Autodesk Fusion 360 part; units mm, degrees
(part 7 of 25)
  arc A2762 (31.8052, 43.4657) -> (31.8052, 43.5293) centre (31.8052, 43.4975) ccw
  arc A2763 (9.9295, 17.8435) -> (9.866, 17.8435) centre (9.8978, 17.8435) ccw
  arc A2764 (11.39, 17.0815) -> (11.3265, 17.0815) centre (11.3582, 17.0815) ccw
  arc A2765 (9.866, 16.7005) -> (9.9295, 16.7005) centre (9.8978, 16.7005) ccw
  arc A2766 (30.353, 44.0055) -> (30.353, 44.6405) centre (30.353, 44.323) ccw
  arc A2767 (32.6942, 43.4657) -> (32.6942, 43.5293) centre (32.6942, 43.4975) ccw
  line L862 (9.5802, 16.7005) -> (10.2152, 16.7005)
  line L863 (10.7232, 17.018) -> (10.7232, 17.3355)
  line L864 (9.5802, 17.5895) -> (9.8977, 17.8435)
  arc A2768 (8.4773, 17.8435) -> (8.4138, 17.8435) centre (8.4456, 17.8435) ccw
  arc A2769 (9.5802, 16.7323) -> (9.5802, 16.6688) centre (9.5802, 16.7005) ccw
  line L865 (10.7232, 17.3355) -> (11.1042, 17.3355)
  line L866 (30.0355, 43.4975) -> (30.0355, 44.6405)
  line L867 (32.3132, 44.6405) -> (32.9482, 44.6405)
  arc A2770 (11.3265, 17.0815) -> (11.39, 17.0815) centre (11.3582, 17.0815) ccw
  arc A2771 (32.2815, 44.1325) -> (32.345, 44.1325) centre (32.3133, 44.1325) ccw
  arc A2772 (8.4138, 16.7005) -> (8.4773, 16.7005) centre (8.4456, 16.7005) ccw
  arc A2773 (30.353, 44.6088) -> (30.353, 44.6723) centre (30.353, 44.6406) ccw
  arc A2774 (32.3132, 44.6723) -> (32.3132, 44.6088) centre (32.3132, 44.6406) ccw
  arc A2775 (32.98, 43.8785) -> (32.9165, 43.8785) centre (32.9483, 43.8785) ccw
  arc A2776 (8.4455, 17.8753) -> (8.4455, 17.8118) centre (8.4455, 17.8436) ccw
  arc A2777 (32.9165, 43.8785) -> (32.98, 43.8785) centre (32.9483, 43.8785) ccw
  arc A2778 (32.6942, 44.1643) -> (32.6942, 44.1007) centre (32.6942, 44.1325) ccw
  arc A2779 (8.4455, 17.2402) -> (8.4455, 17.1768) centre (8.4455, 17.2085) ccw
  arc A2780 (9.9175, 17.8187) -> (9.8779, 17.8683) centre (9.8977, 17.8435) ccw
  arc A2781 (10.7232, 17.3672) -> (10.7232, 17.3038) centre (10.7232, 17.3355) ccw
  arc A2782 (32.3132, 43.5293) -> (32.3132, 43.4657) centre (32.3132, 43.4975) ccw
  arc A2783 (10.755, 17.018) -> (10.6915, 17.018) centre (10.7233, 17.018) ccw
  arc A2784 (10.755, 17.3355) -> (10.6915, 17.3355) centre (10.7233, 17.3355) ccw
  line L868 (8.4455, 16.7005) -> (8.4455, 17.8435)
  arc A2785 (32.9482, 43.8785) -> (32.6942, 44.1325) centre (32.6942, 43.8785) ccw
  line L869 (8.763, 17.2085) -> (8.4455, 17.2085)
  arc A2786 (32.9482, 44.6088) -> (32.9482, 44.6723) centre (32.9482, 44.6406) ccw
  line L870 (32.6942, 44.1325) -> (32.3132, 44.1325)
  line L871 (32.9482, 43.7515) -> (32.9482, 43.8785)
  line L872 (8.4455, 17.8435) -> (8.763, 17.8435)
  arc A2787 (8.763, 17.8753) -> (8.763, 17.8118) centre (8.763, 17.8436) ccw
  arc A2788 (10.2152, 16.6688) -> (10.2152, 16.7323) centre (10.2152, 16.7005) ccw
  arc A2789 (32.3132, 44.1643) -> (32.3132, 44.1007) centre (32.3132, 44.1325) ccw
  arc A2790 (11.3265, 17.018) -> (11.39, 17.018) centre (11.3582, 17.018) ccw
  arc A2791 (32.6942, 44.1007) -> (32.6942, 44.1643) centre (32.6942, 44.1325) ccw
  arc A2792 (10.7232, 17.018) -> (11.3582, 17.018) centre (11.0407, 17.018) ccw
  arc A2793 (8.763, 17.2402) -> (8.763, 17.1768) centre (8.763, 17.2085) ccw
  arc A2794 (8.763, 17.8118) -> (8.763, 17.8753) centre (8.763, 17.8436) ccw
  arc A2795 (11.2312, 17.8118) -> (11.2312, 17.8753) centre (11.2312, 17.8436) ccw
  line L873 (9.8977, 17.8435) -> (9.8977, 16.7005)
  arc A2796 (9.0521, 16.6863) -> (9.1089, 16.7147) centre (9.0805, 16.7005) ccw
  arc A2797 (82.4992, 5.1474) -> (82.5296, 5.2031) centre (82.5144, 5.1753) ccw
  arc A2798 (82.3595, 18.6055) -> (82.6135, 18.8595) centre (82.3595, 18.8595) ccw
  arc A2799 (82.4713, 19.0539) -> (82.5017, 19.1096) centre (82.4865, 19.0817) ccw
  arc A2800 (83.4326, 19.7168) -> (83.4327, 19.7802) centre (83.4326, 19.7485) ccw
  arc A2801 (83.0915, 5.6128) -> (83.1312, 5.5632) centre (83.1114, 5.588) ccw
  arc A2802 (82.5309, 19.6279) -> (82.5691, 19.6786) centre (82.55, 19.6532) ccw
  arc A2803 (82.1804, 5.3936) -> (82.15, 5.3379) centre (82.1652, 5.3657) ccw
  arc A2804 (82.5026, 19.1091) -> (82.4704, 19.0544) centre (82.4865, 19.0817) ccw
  line L874 (83.1113, 5.588) -> (83.4288, 5.842)
  arc A2805 (82.0699, 5.588) -> (82.0064, 5.588) centre (82.0382, 5.588) ccw
  line L875 (82.5144, 5.1753) -> (82.1652, 5.3658)
  arc A2806 (82.0064, 4.8578) -> (82.3874, 4.699) centre (82.3875, 5.2356) ccw
  arc A2807 (83.7463, 4.6673) -> (83.7463, 4.7307) centre (83.7463, 4.699) ccw
  arc A2808 (82.3595, 18.6372) -> (82.3595, 18.5738) centre (82.3595, 18.6055) ccw
  arc A2809 (83.4487, 5.8172) -> (83.409, 5.8668) centre (83.4289, 5.842) ccw
  arc A2810 (82.3874, 4.7307) -> (82.3874, 4.6673) centre (82.3874, 4.699) ccw
  arc A2811 (83.0592, 18.6261) -> (83.1076, 18.5849) centre (83.0834, 18.6055) ccw
  arc A2812 (82.6097, 4.953) -> (82.6732, 4.953) centre (82.6414, 4.953) ccw
  arc A2813 (82.2643, 19.7485) -> (82.0102, 19.4945) centre (82.2643, 19.4944) ccw
  arc A2814 (83.4327, 19.7802) -> (83.4327, 19.7168) centre (83.4327, 19.7485) ccw
  arc A2815 (83.7501, 19.4628) -> (83.6867, 19.4627) centre (83.7184, 19.4628) ccw
  arc A2816 (83.3971, 4.699) -> (83.4606, 4.699) centre (83.4288, 4.699) ccw
  arc A2817 (82.5779, 5.7468) -> (82.2922, 5.842) centre (82.2923, 5.3659) ccw
  arc A2818 (82.6453, 18.8595) -> (82.5817, 18.8595) centre (82.6135, 18.8595) ccw
  arc A2819 (82.55, 19.6532) -> (82.2643, 19.7485) centre (82.2642, 19.2724) ccw
  arc A2820 (82.2643, 19.7168) -> (82.2643, 19.7802) centre (82.2643, 19.7485) ccw
  line L876 (83.6232, 19.2405) -> (83.0834, 18.6055)
  arc A2821 (83.6473, 19.2199) -> (83.599, 19.2611) centre (83.6232, 19.2405) ccw
  arc A2822 (83.0834, 18.6372) -> (83.0834, 18.5738) centre (83.0834, 18.6055) ccw
  arc A2823 (82.1211, 19.2449) -> (82.1534, 19.2996) centre (82.1372, 19.2723) ccw
  arc A2824 (82.3595, 18.5738) -> (82.3595, 18.6372) centre (82.3595, 18.6055) ccw
  arc A2825 (83.0532, 19.5043) -> (83.1136, 19.4847) centre (83.0834, 19.4945) ccw
  arc A2826 (82.1491, 5.3384) -> (82.1813, 5.3931) centre (82.1652, 5.3658) ccw
  line L877 (83.0834, 18.6055) -> (83.7184, 18.6055)
  arc A2827 (82.029, 4.8801) -> (81.9839, 4.8354) centre (82.0065, 4.8577) ccw
  arc A2828 (82.2922, 5.8738) -> (82.2922, 5.8103) centre (82.2922, 5.842) ccw
  arc A2829 (83.4606, 5.842) -> (83.3971, 5.842) centre (83.4288, 5.842) ccw
  arc A2830 (10.6915, 17.018) -> (10.755, 17.018) centre (10.7233, 17.018) ccw
  arc A2831 (82.6732, 4.953) -> (82.6097, 4.953) centre (82.6414, 4.953) ccw
  arc A2832 (82.0064, 5.588) -> (82.0699, 5.588) centre (82.0382, 5.588) ccw
  arc A2833 (83.6013, 19.2635) -> (83.645, 19.2175) centre (83.6231, 19.2405) ccw
  arc A2834 (82.2642, 19.7802) -> (82.2643, 19.7168) centre (82.2643, 19.7485) ccw
  arc A2835 (83.7184, 18.5738) -> (83.7184, 18.6372) centre (83.7184, 18.6055) ccw
  line L878 (83.1113, 4.699) -> (83.7463, 4.699)
  arc A2836 (82.0382, 5.588) -> (82.1652, 5.3658) centre (82.2961, 5.588) ccw
  arc A2837 (82.001, 18.7866) -> (81.956, 18.7419) centre (81.9785, 18.7643) ccw
  arc A2838 (83.4327, 19.7485) -> (83.0834, 19.4945) centre (83.4327, 19.3814) ccw
  arc A2839 (81.9785, 19.4945) -> (82.042, 19.4945) centre (82.0103, 19.4945) ccw
  arc A2840 (82.5306, 5.2026) -> (82.4983, 5.1479) centre (82.5145, 5.1753) ccw
  arc A2841 (82.2922, 5.842) -> (82.0382, 5.588) centre (82.2922, 5.588) ccw
  line L879 (83.4288, 5.842) -> (83.4288, 4.699)
  arc A2842 (82.5589, 5.7214) -> (82.597, 5.7721) centre (82.5779, 5.7468) ccw
  arc A2843 (11.1042, 17.3672) -> (11.1042, 17.3038) centre (11.1042, 17.3355) ccw
  arc A2844 (82.3874, 4.6673) -> (82.3874, 4.7307) centre (82.3874, 4.699) ccw
  arc A2845 (81.9785, 18.7643) -> (82.3595, 18.6055) centre (82.3596, 19.1421) ccw
  arc A2846 (11.1042, 17.3038) -> (11.1042, 17.3672) centre (11.1042, 17.3355) ccw
  arc A2847 (83.6867, 19.4627) -> (83.7502, 19.4627) centre (83.7185, 19.4627) ccw
  arc A2848 (11.2312, 17.8435) -> (10.7232, 17.3355) centre (11.2312, 17.3355) ccw
  arc A2849 (11.3582, 17.0815) -> (11.1042, 17.3355) centre (11.1042, 17.0815) ccw
  arc A2850 (82.2922, 5.8103) -> (82.2922, 5.8738) centre (82.2922, 5.842) ccw
  arc A2851 (82.6414, 4.953) -> (82.5144, 5.1753) centre (82.3834, 4.953) ccw
  arc A2852 (83.1113, 4.7307) -> (83.1113, 4.6673) centre (83.1113, 4.699) ccw
  line L880 (82.4865, 19.0817) -> (82.1373, 19.2722)
  arc A2853 (15.326, 27.5496) -> (15.281, 27.5049) centre (15.3035, 27.5273) ccw
  arc A2854 (15.875, 28.4163) -> (15.5893, 28.5115) centre (15.5894, 28.0354) ccw
  line L881 (16.7005, 28.5115) -> (17.0815, 28.5115)
  arc A2855 (15.4461, 28.0079) -> (15.4784, 28.0626) centre (15.4623, 28.0352) ccw
  arc A2856 (16.4782, 27.6225) -> (16.4148, 27.6225) centre (16.4465, 27.6225) ccw
  arc A2857 (17.6078, 28.2823) -> (17.6474, 28.2327) centre (17.6276, 28.2575) ccw
  line L882 (20.3073, 36.1315) -> (20.6248, 36.3855)
  arc A2858 (16.891, 28.0353) -> (16.891, 27.9718) centre (16.891, 28.0036) ccw
  line L883 (17.6276, 27.3685) -> (18.2626, 27.3685)
  arc A2859 (17.0815, 27.3368) -> (17.0815, 27.4002) centre (17.0815, 27.3685) ccw
  arc A2860 (15.9068, 27.6225) -> (15.9703, 27.6225) centre (15.9386, 27.6225) ccw
  arc A2861 (16.7005, 28.5115) -> (16.4465, 28.2575) centre (16.7005, 28.2575) ccw
  arc A2862 (15.4775, 28.0631) -> (15.447, 28.0074) centre (15.4622, 28.0353) ccw
  arc A2863 (17.0815, 28.4798) -> (17.0815, 28.5433) centre (17.0815, 28.5115) ccw
  arc A2864 (82.042, 19.4945) -> (81.9785, 19.4945) centre (82.0103, 19.4945) ccw
  arc A2865 (82.6135, 18.8595) -> (82.4865, 19.0817) centre (82.3556, 18.8595) ccw
  arc A2866 (82.1525, 19.3001) -> (82.122, 19.2444) centre (82.1372, 19.2723) ccw
  arc A2867 (16.4782, 28.2575) -> (16.4148, 28.2575) centre (16.4465, 28.2575) ccw
  arc A2868 (15.5892, 28.5433) -> (15.5893, 28.4798) centre (15.5893, 28.5115) ccw
  arc A2869 (17.0815, 27.9718) -> (17.0815, 28.0353) centre (17.0815, 28.0036) ccw
  arc A2870 (18.2626, 27.3368) -> (18.2626, 27.4002) centre (18.2626, 27.3685) ccw
  line L884 (20.6248, 36.3855) -> (20.6248, 35.2425)
  arc A2871 (15.3035, 27.5273) -> (15.6845, 27.3685) centre (15.6846, 27.9051) ccw
  arc A2872 (16.7005, 27.4002) -> (16.7005, 27.3368) centre (16.7005, 27.3685) ccw
  arc A2873 (15.3035, 28.2575) -> (15.367, 28.2575) centre (15.3353, 28.2575) ccw
  arc A2874 (82.0102, 19.4945) -> (82.1373, 19.2722) centre (82.2682, 19.4945) ccw
  line L885 (16.891, 28.0035) -> (17.0815, 28.0035)
  arc A2875 (15.5893, 28.4798) -> (15.5893, 28.5433) centre (15.5893, 28.5115) ccw
  arc A2876 (82.5817, 18.8595) -> (82.6453, 18.8595) centre (82.6135, 18.8595) ccw
  arc A2877 (15.6845, 27.3368) -> (15.6845, 27.4002) centre (15.6845, 27.3685) ccw
  arc A2878 (83.6232, 19.2405) -> (83.7184, 19.4627) centre (83.4116, 19.4626) ccw
  line L886 (19.558, 35.2425) -> (19.558, 36.3855)
  line L887 (16.4465, 27.6225) -> (16.4465, 28.2575)
  line L888 (17.0815, 28.0035) -> (17.0815, 27.3685)
  arc A2879 (19.5263, 35.2425) -> (19.5897, 35.2425) centre (19.558, 35.2425) ccw
  arc A2880 (20.6446, 36.3607) -> (20.605, 36.4103) centre (20.6248, 36.3855) ccw
  arc A2881 (20.2875, 36.1563) -> (20.3271, 36.1067) centre (20.3073, 36.1315) ccw
  arc A2882 (16.4465, 27.6225) -> (16.7005, 27.3685) centre (16.7005, 27.6225) ccw
  arc A2883 (15.9703, 27.6225) -> (15.9068, 27.6225) centre (15.9386, 27.6225) ccw
  arc A2884 (15.8559, 28.3909) -> (15.8941, 28.4416) centre (15.875, 28.4163) ccw
  arc A2885 (83.7184, 19.4627) -> (83.4327, 19.7485) centre (83.4326, 19.4627) ccw
  arc A2886 (17.9134, 27.3685) -> (17.9768, 27.3685) centre (17.9451, 27.3685) ccw
  arc A2887 (16.7005, 27.3368) -> (16.7005, 27.4002) centre (16.7005, 27.3685) ccw
  arc A2888 (15.5893, 28.5115) -> (15.3353, 28.2575) centre (15.5893, 28.2575) ccw
  arc A2889 (17.9649, 28.4867) -> (17.9253, 28.5363) centre (17.9451, 28.5115) ccw
  arc A2890 (20.6565, 36.3855) -> (20.5931, 36.3855) centre (20.6248, 36.3855) ccw
  line L889 (17.9451, 28.5115) -> (17.9451, 27.3685)
  line L890 (19.2405, 36.3855) -> (19.8755, 36.3855)
  arc A2891 (16.7005, 28.4798) -> (16.7005, 28.5433) centre (16.7005, 28.5115) ccw
  arc A2892 (16.4148, 27.6225) -> (16.4782, 27.6225) centre (16.4465, 27.6225) ccw
  arc A2893 (17.0498, 27.3685) -> (17.1133, 27.3685) centre (17.0816, 27.3685) ccw
  arc A2894 (16.4148, 28.2575) -> (16.4782, 28.2575) centre (16.4465, 28.2575) ccw
  line L891 (17.0815, 27.3685) -> (16.7005, 27.3685)
  arc A2895 (15.6845, 27.4002) -> (15.6845, 27.3368) centre (15.6845, 27.3685) ccw
  arc A2896 (15.8276, 27.8721) -> (15.7954, 27.8174) centre (15.8115, 27.8448) ccw
  arc A2897 (15.3353, 28.2575) -> (15.4623, 28.0353) centre (15.5932, 28.2575) ccw
  arc A2898 (15.367, 28.2575) -> (15.3035, 28.2575) centre (15.3353, 28.2575) ccw
  line L892 (15.8115, 27.8448) -> (15.4623, 28.0353)
  arc A2899 (15.7963, 27.8169) -> (15.8267, 27.8726) centre (15.8115, 27.8448) ccw
  arc A2900 (17.1133, 28.0035) -> (17.0498, 28.0035) centre (17.0816, 28.0035) ccw
  arc A2901 (15.9385, 27.6225) -> (15.8115, 27.8448) centre (15.6805, 27.6225) ccw
  arc A2902 (16.7005, 28.5433) -> (16.7005, 28.4798) centre (16.7005, 28.5115) ccw
  line L893 (17.6276, 28.2575) -> (17.9451, 28.5115)
  arc A2903 (15.6845, 27.3685) -> (15.9385, 27.6225) centre (15.6845, 27.6225) ccw
  arc A2904 (17.6276, 27.4002) -> (17.6276, 27.3368) centre (17.6276, 27.3685) ccw
  arc A2905 (20.5931, 35.2425) -> (20.6565, 35.2425) centre (20.6248, 35.2425) ccw
  line L894 (20.3073, 35.2425) -> (20.9423, 35.2425)
  arc A2906 (17.9768, 28.5115) -> (17.9134, 28.5115) centre (17.9451, 28.5115) ccw
  arc A2907 (19.2405, 36.4173) -> (19.2405, 36.3537) centre (19.2405, 36.3855) ccw
  arc A2908 (19.5897, 36.3855) -> (19.5263, 36.3855) centre (19.558, 36.3855) ccw
  arc A2909 (20.3073, 35.2743) -> (20.3073, 35.2107) centre (20.3073, 35.2425) ccw
  arc A2910 (20.9423, 35.2107) -> (20.9423, 35.2743) centre (20.9423, 35.2425) ccw
  arc A2911 (19.8755, 36.3537) -> (19.8755, 36.4173) centre (19.8755, 36.3855) ccw
sketch "Botton Trace" plane through (0, 0, 0) normal (0, 0, 1) x (1, 0, 0)
  arc A0 (82.7578, 33.1788) -> (82.7578, 32.8613) centre (82.7578, 33.0201) ccw
  arc A1 (15.6337, 33.8137) -> (15.6337, 33.4963) centre (15.6337, 33.655) ccw
  arc A2 (82.4468, 33.8137) -> (82.4468, 33.4963) centre (82.4468, 33.655) ccw
  arc A3 (66.04, 33.1788) -> (66.04, 32.8613) centre (66.04, 33.0201) ccw
  arc A4 (81.28, 32.8613) -> (81.28, 33.1788) centre (81.28, 33.0201) ccw
  arc A5 (66.04, 33.4963) -> (66.04, 33.8137) centre (66.04, 33.655) ccw
  arc A6 (0.7747, 33.8137) -> (0.7747, 33.4963) centre (0.7747, 33.655) ccw
  arc A7 (52.818, 33.8137) -> (52.818, 33.4963) centre (52.818, 33.655) ccw
  arc A8 (15.7861, 33.4963) -> (15.7861, 33.8137) centre (15.7861, 33.655) ccw
  arc A9 (71.8947, 32.8613) -> (71.8947, 33.1788) centre (71.8947, 33.0201) ccw
  arc A10 (81.28, 33.8137) -> (81.28, 33.4963) centre (81.28, 33.655) ccw
  arc A11 (35.9156, 33.8137) -> (35.9156, 33.4963) centre (35.9156, 33.655) ccw
  arc A12 (39.1736, 33.4963) -> (39.1736, 33.8137) centre (39.1736, 33.655) ccw
  arc A13 (11.289, 33.8137) -> (11.289, 33.4963) centre (11.289, 33.655) ccw
  arc A14 (52.2859, 33.1788) -> (52.2859, 32.8613) centre (52.2859, 33.0201) ccw
  arc A15 (33.2611, 32.8613) -> (33.2611, 33.1788) centre (33.2611, 33.0201) ccw
  arc A16 (84.2253, 32.8613) -> (84.2253, 33.1788) centre (84.2253, 33.0201) ccw
  arc A17 (17.7419, 33.8137) -> (17.7419, 33.4963) centre (17.7419, 33.655) ccw
  arc A18 (35.3189, 33.1788) -> (35.3189, 32.8613) centre (35.3189, 33.0201) ccw
  arc A19 (31.002, 33.4963) -> (31.002, 33.8137) centre (31.002, 33.655) ccw
  arc A20 (48.6064, 33.1788) -> (48.6064, 32.8613) centre (48.6064, 33.0201) ccw
  arc A21 (17.7419, 33.1788) -> (17.7419, 32.8613) centre (17.7419, 33.0201) ccw
  arc A22 (49.3141, 32.8613) -> (49.3141, 33.1788) centre (49.3141, 33.0201) ccw
  arc A23 (54.9021, 32.8613) -> (54.9021, 33.1788) centre (54.9021, 33.0201) ccw
  arc A24 (84.2253, 33.4963) -> (84.2253, 33.8137) centre (84.2253, 33.655) ccw
  arc A25 (28.2956, 34.4487) -> (28.2956, 34.1313) centre (28.2956, 34.29) ccw
  arc A26 (0.7747, 35.0838) -> (0.7747, 34.7663) centre (0.7747, 34.925) ccw
  line L0 (61.7097, 34.29) -> (62.7503, 34.29)
  arc A27 (84.2253, 34.1313) -> (84.2253, 34.4487) centre (84.2253, 34.29) ccw
  arc A28 (72.517, 34.1313) -> (72.517, 34.4487) centre (72.517, 34.29) ccw
  arc A29 (61.7097, 34.4487) -> (61.7097, 34.1313) centre (61.7097, 34.29) ccw
  arc A30 (17.7419, 34.4487) -> (17.7419, 34.1313) centre (17.7419, 34.29) ccw
  arc A31 (79.7179, 34.4487) -> (79.7179, 34.1313) centre (79.7179, 34.29) ccw
  arc A32 (25.0444, 34.1313) -> (25.0444, 34.4487) centre (25.0444, 34.29) ccw
  arc A33 (56.974, 35.0838) -> (56.974, 34.7663) centre (56.974, 34.925) ccw
  arc A34 (57.1337, 34.4487) -> (57.1337, 34.1313) centre (57.1337, 34.29) ccw
  arc A35 (12.6332, 34.7663) -> (12.6332, 35.0838) centre (12.6332, 34.925) ccw
  arc A36 (60.2103, 34.1313) -> (60.2103, 34.4487) centre (60.2103, 34.29) ccw
  arc A37 (15.613, 34.4487) -> (15.613, 34.1313) centre (15.613, 34.29) ccw
  arc A38 (30.367, 34.1313) -> (30.367, 34.4487) centre (30.367, 34.29) ccw
  arc A39 (54.6263, 34.1313) -> (54.6263, 34.4487) centre (54.6263, 34.29) ccw
  arc A40 (39.8086, 34.1313) -> (39.8086, 34.4487) centre (39.8086, 34.29) ccw
  arc A41 (49.9686, 34.1313) -> (49.9686, 34.4487) centre (49.9686, 34.29) ccw
  arc A42 (35.9156, 34.4487) -> (35.9156, 34.1313) centre (35.9156, 34.29) ccw
  arc A43 (1.0423, 34.7663) -> (1.0423, 35.0838) centre (1.0423, 34.925) ccw
  arc A44 (53.453, 34.4487) -> (53.453, 34.1313) centre (53.453, 34.29) ccw
  arc A45 (62.7503, 34.1313) -> (62.7503, 34.4487) centre (62.7503, 34.29) ccw
  arc A46 (39.0236, 32.8613) -> (39.0236, 33.1788) centre (39.0236, 33.0201) ccw
  arc A47 (81.28, 33.1788) -> (81.28, 32.8613) centre (81.28, 33.0201) ccw
  arc A48 (79.7179, 35.0838) -> (79.7179, 34.7663) centre (79.7179, 34.925) ccw
  arc A49 (41.4714, 34.4487) -> (41.4714, 34.1313) centre (41.4714, 34.29) ccw
  arc A50 (72.517, 34.7663) -> (72.517, 35.0838) centre (72.517, 34.925) ccw
  arc A51 (54.088, 35.0838) -> (54.088, 34.7663) centre (54.088, 34.925) ccw
  arc A52 (10.654, 34.4487) -> (10.654, 34.1313) centre (10.654, 34.29) ccw
  arc A53 (84.2253, 34.7663) -> (84.2253, 35.0838) centre (84.2253, 34.925) ccw
  arc A54 (12.3063, 33.4963) -> (12.3063, 33.8137) centre (12.3063, 33.655) ccw
  arc A55 (15.7861, 34.7663) -> (15.7861, 35.0838) centre (15.7861, 34.925) ccw
  arc A56 (66.04, 32.8613) -> (66.04, 33.1788) centre (66.04, 33.0201) ccw
  arc A57 (25.0444, 33.4963) -> (25.0444, 33.8137) centre (25.0444, 33.655) ccw
  arc A58 (15.7861, 34.1313) -> (15.7861, 34.4487) centre (15.7861, 34.29) ccw
  arc A59 (25.6411, 32.8613) -> (25.6411, 33.1788) centre (25.6411, 33.0201) ccw
  arc A60 (56.8579, 33.1788) -> (56.8579, 32.8613) centre (56.8579, 33.0201) ccw
  arc A61 (0.9017, 34.1313) -> (0.9017, 34.4487) centre (0.9017, 34.29) ccw
  arc A62 (29.5021, 36.6713) -> (29.5021, 36.9887) centre (29.5021, 36.83) ccw
  arc A63 (72.214, 36.3537) -> (72.214, 36.0363) centre (72.214, 36.195) ccw
  arc A64 (4.5252, 35.7188) -> (4.5252, 35.4013) centre (4.5252, 35.5601) ccw
  arc A65 (15.7861, 35.4013) -> (15.7861, 35.7188) centre (15.7861, 35.5601) ccw
  arc A66 (6.6508, 35.4013) -> (6.6508, 35.7188) centre (6.6508, 35.5601) ccw
  arc A67 (72.517, 35.4013) -> (72.517, 35.7188) centre (72.517, 35.5601) ccw
  arc A68 (17.7419, 35.7188) -> (17.7419, 35.4013) centre (17.7419, 35.5601) ccw
  arc A69 (25.6411, 35.4013) -> (25.6411, 35.7188) centre (25.6411, 35.5601) ccw
  arc A70 (72.517, 36.0363) -> (72.517, 36.3537) centre (72.517, 36.195) ccw
  arc A71 (25.0444, 34.7663) -> (25.0444, 35.0838) centre (25.0444, 34.925) ccw
  arc A72 (51.322, 34.7663) -> (51.322, 35.0838) centre (51.322, 34.925) ccw
  arc A73 (27.6989, 36.9887) -> (27.6989, 36.6713) centre (27.6989, 36.83) ccw
  arc A74 (17.7419, 35.0838) -> (17.7419, 34.7663) centre (17.7419, 34.925) ccw
  arc A75 (29.732, 34.7663) -> (29.732, 35.0838) centre (29.732, 34.925) ccw
  arc A76 (64.2497, 34.4487) -> (64.2497, 34.1313) centre (64.2497, 34.29) ccw
  arc A77 (52.592, 36.0363) -> (52.592, 36.3537) centre (52.592, 36.195) ccw
  arc A78 (0.7747, 35.7188) -> (0.7747, 35.4013) centre (0.7747, 35.5601) ccw
  arc A79 (15.3068, 35.0838) -> (15.3068, 34.7663) centre (15.3068, 34.925) ccw
  arc A80 (35.9156, 35.0838) -> (35.9156, 34.7663) centre (35.9156, 34.925) ccw
  arc A81 (11.0836, 36.6713) -> (11.0836, 36.9887) centre (11.0836, 36.83) ccw
  arc A82 (84.2253, 35.4013) -> (84.2253, 35.7188) centre (84.2253, 35.5601) ccw
  arc A83 (14.3164, 36.9887) -> (14.3164, 36.6713) centre (14.3164, 36.83) ccw
  arc A84 (29.5021, 35.4013) -> (29.5021, 35.7188) centre (29.5021, 35.5601) ccw
  arc A85 (1.5708, 35.4013) -> (1.5708, 35.7188) centre (1.5708, 35.5601) ccw
  arc A86 (28.2956, 35.0838) -> (28.2956, 34.7663) centre (28.2956, 34.925) ccw
  arc A87 (29.5021, 36.0363) -> (29.5021, 36.3537) centre (29.5021, 36.195) ccw
  arc A88 (15.7861, 36.0363) -> (15.7861, 36.3537) centre (15.7861, 36.195) ccw
  arc A89 (10.1337, 35.0838) -> (10.1337, 34.7663) centre (10.1337, 34.925) ccw
  arc A90 (54.786, 34.7663) -> (54.786, 35.0838) centre (54.786, 34.925) ccw
  arc A91 (12.327, 34.1313) -> (12.327, 34.4487) centre (12.327, 34.29) ccw
  arc A92 (12.3536, 35.4013) -> (12.3536, 35.7188) centre (12.3536, 35.5601) ccw
  arc A93 (25.6921, 36.0363) -> (25.6921, 36.3537) centre (25.6921, 36.195) ccw
  arc A94 (17.7419, 36.3537) -> (17.7419, 36.0363) centre (17.7419, 36.195) ccw
  arc A95 (79.7179, 35.7188) -> (79.7179, 35.4013) centre (79.7179, 35.5601) ccw
  arc A96 (27.6989, 35.7188) -> (27.6989, 35.4013) centre (27.6989, 35.5601) ccw
  arc A97 (25.6411, 36.6713) -> (25.6411, 36.9887) centre (25.6411, 36.83) ccw
  arc A98 (15.113, 35.7188) -> (15.113, 35.4013) centre (15.113, 35.5601) ccw
  arc A99 (0.7747, 34.4487) -> (0.7747, 34.1313) centre (0.7747, 34.29) ccw
  arc A100 (27.6479, 36.3537) -> (27.6479, 36.0363) centre (27.6479, 36.195) ccw
  arc A101 (33.2611, 36.6713) -> (33.2611, 36.9887) centre (33.2611, 36.83) ccw
  arc A102 (0.7747, 36.3537) -> (0.7747, 36.0363) centre (0.7747, 36.195) ccw
  arc A103 (31.4579, 36.3537) -> (31.4579, 36.0363) centre (31.4579, 36.195) ccw
  arc A104 (84.2253, 36.0363) -> (84.2253, 36.3537) centre (84.2253, 36.195) ccw
  arc A105 (31.4579, 36.9887) -> (31.4579, 36.6713) centre (31.4579, 36.83) ccw
  arc A106 (35.3189, 36.9887) -> (35.3189, 36.6713) centre (35.3189, 36.83) ccw
  arc A107 (17.7419, 36.9887) -> (17.7419, 36.6713) centre (17.7419, 36.83) ccw
  arc A108 (51.6314, 36.9887) -> (51.6314, 36.6713) centre (51.6314, 36.83) ccw
  arc A109 (51.957, 35.4013) -> (51.957, 35.7188) centre (51.957, 35.5601) ccw
  arc A110 (79.7179, 36.3537) -> (79.7179, 36.0363) centre (79.7179, 36.195) ccw
  arc A111 (31.863, 35.7188) -> (31.863, 35.4013) centre (31.863, 35.5601) ccw
  arc A112 (9.6052, 35.7188) -> (9.6052, 35.4013) centre (9.6052, 35.5601) ccw
  arc A113 (72.214, 37.6238) -> (72.214, 37.3063) centre (72.214, 37.4651) ccw
  arc A114 (20.32, 37.9413) -> (20.32, 38.2587) centre (20.32, 38.1) ccw
  arc A115 (39.8086, 36.6713) -> (39.8086, 36.9887) centre (39.8086, 36.83) ccw
  arc A116 (33.2611, 35.4013) -> (33.2611, 35.7188) centre (33.2611, 35.5601) ccw
  arc A117 (0.7747, 36.9887) -> (0.7747, 36.6713) centre (0.7747, 36.83) ccw
  arc A118 (31.4579, 37.6238) -> (31.4579, 37.3063) centre (31.4579, 37.4651) ccw
  arc A119 (84.2253, 36.6713) -> (84.2253, 36.9887) centre (84.2253, 36.83) ccw
  arc A120 (18.6006, 37.3063) -> (18.6006, 37.6238) centre (18.6006, 37.4651) ccw
  arc A121 (79.7179, 36.9887) -> (79.7179, 36.6713) centre (79.7179, 36.83) ccw
  arc A122 (17.7419, 37.6238) -> (17.7419, 37.3063) centre (17.7419, 37.4651) ccw
  arc A123 (25.0444, 37.3063) -> (25.0444, 37.6238) centre (25.0444, 37.4651) ccw
  arc A124 (0.7747, 38.2587) -> (0.7747, 37.9413) centre (0.7747, 38.1) ccw
  arc A125 (3.4636, 37.9413) -> (3.4636, 38.2587) centre (3.4636, 38.1) ccw
  arc A126 (28.2956, 37.6238) -> (28.2956, 37.3063) centre (28.2956, 37.4651) ccw
  arc A127 (13.6814, 37.6238) -> (13.6814, 37.3063) centre (13.6814, 37.4651) ccw
  arc A128 (39.1736, 37.3063) -> (39.1736, 37.6238) centre (39.1736, 37.4651) ccw
  arc A129 (15.7861, 36.6713) -> (15.7861, 36.9887) centre (15.7861, 36.83) ccw
  arc A130 (17.7419, 38.2587) -> (17.7419, 37.9413) centre (17.7419, 38.1) ccw
  arc A131 (72.517, 36.6713) -> (72.517, 36.9887) centre (72.517, 36.83) ccw
  arc A132 (20.32, 37.6238) -> (20.32, 37.3063) centre (20.32, 37.4651) ccw
  arc A133 (35.3189, 35.7188) -> (35.3189, 35.4013) centre (35.3189, 35.5601) ccw
  arc A134 (49.9686, 36.6713) -> (49.9686, 36.9887) centre (49.9686, 36.83) ccw
  arc A135 (4.0986, 37.3063) -> (4.0986, 37.6238) centre (4.0986, 37.4651) ccw
  arc A136 (22.0394, 37.6238) -> (22.0394, 37.3063) centre (22.0394, 37.4651) ccw
  arc A137 (11.7186, 36.0363) -> (11.7186, 36.3537) centre (11.7186, 36.195) ccw
  arc A138 (20.32, 37.3063) -> (20.32, 37.6238) centre (20.32, 37.4651) ccw
  arc A139 (20.32, 38.2587) -> (20.32, 37.9413) centre (20.32, 38.1) ccw
  arc A140 (15.7861, 37.9413) -> (15.7861, 38.2587) centre (15.7861, 38.1) ccw
  arc A141 (72.3737, 36.9887) -> (72.3737, 36.6713) centre (72.3737, 36.83) ccw
  arc A142 (41.4714, 36.9887) -> (41.4714, 36.6713) centre (41.4714, 36.83) ccw
  arc A143 (15.7861, 37.3063) -> (15.7861, 37.6238) centre (15.7861, 37.4651) ccw
  arc A144 (53.227, 36.6713) -> (53.227, 36.9887) centre (53.227, 36.83) ccw
  arc A145 (54.723, 35.7188) -> (54.723, 35.4013) centre (54.723, 35.5601) ccw
  arc A146 (14.9442, 36.3537) -> (14.9442, 36.0363) centre (14.9442, 36.195) ccw
  arc A147 (13.0464, 38.2587) -> (13.0464, 37.9413) centre (13.0464, 38.1) ccw
  arc A148 (25.0444, 37.9413) -> (25.0444, 38.2587) centre (25.0444, 38.1) ccw
  arc A149 (29.5021, 37.9413) -> (29.5021, 38.2587) centre (29.5021, 38.1) ccw
  arc A150 (0.7747, 37.6238) -> (0.7747, 37.3063) centre (0.7747, 37.4651) ccw
  arc A151 (49.3336, 38.5763) -> (49.3336, 38.8937) centre (49.3336, 38.735) ccw
  arc A152 (84.2253, 38.5763) -> (84.2253, 38.8937) centre (84.2253, 38.735) ccw
  arc A153 (0.7747, 39.5288) -> (0.7747, 39.2113) centre (0.7747, 39.37) ccw
  arc A154 (72.517, 38.5763) -> (72.517, 38.8937) centre (72.517, 38.735) ccw
  arc A155 (2.8286, 38.5763) -> (2.8286, 38.8937) centre (2.8286, 38.735) ccw
  arc A156 (18.6006, 38.5763) -> (18.6006, 38.8937) centre (18.6006, 38.735) ccw
  arc A157 (79.7179, 38.2587) -> (79.7179, 37.9413) centre (79.7179, 38.1) ccw
  arc A158 (15.7861, 38.5763) -> (15.7861, 38.8937) centre (15.7861, 38.735) ccw
  arc A159 (12.4114, 38.8937) -> (12.4114, 38.5763) centre (12.4114, 38.735) ccw
  arc A160 (2.1936, 39.2113) -> (2.1936, 39.5288) centre (2.1936, 39.37) ccw
  arc A161 (37.578, 37.6238) -> (37.578, 37.3063) centre (37.578, 37.4651) ccw
  arc A162 (49.3336, 37.3063) -> (49.3336, 37.6238) centre (49.3336, 37.4651) ccw
  arc A163 (17.7419, 38.8937) -> (17.7419, 38.5763) centre (17.7419, 38.735) ccw
  arc A164 (21.7972, 39.5288) -> (21.7972, 39.2113) centre (21.7972, 39.37) ccw
  arc A165 (28.2956, 38.8937) -> (28.2956, 38.5763) centre (28.2956, 38.735) ccw
  arc A166 (42.2564, 38.2587) -> (42.2564, 37.9413) centre (42.2564, 38.1) ccw
  arc A167 (38.213, 38.2587) -> (38.213, 37.9413) centre (38.213, 38.1) ccw
  arc A168 (39.1541, 37.9413) -> (39.1541, 38.2587) centre (39.1541, 38.1) ccw
  arc A169 (28.2956, 38.2587) -> (28.2956, 37.9413) centre (28.2956, 38.1) ccw
  arc A170 (27.6989, 39.5288) -> (27.6989, 39.2113) centre (27.6989, 39.37) ccw
  arc A171 (18.8428, 39.2113) -> (18.8428, 39.5288) centre (18.8428, 39.37) ccw
  arc A172 (84.2253, 37.3063) -> (84.2253, 37.6238) centre (84.2253, 37.4651) ccw
  arc A173 (53.862, 37.3063) -> (53.862, 37.6238) centre (53.862, 37.4651) ccw
  arc A174 (32.6644, 37.3063) -> (32.6644, 37.6238) centre (32.6644, 37.4651) ccw
  arc A175 (33.2611, 39.2113) -> (33.2611, 39.5288) centre (33.2611, 39.37) ccw
  arc A176 (22.0394, 38.8937) -> (22.0394, 38.5763) centre (22.0394, 38.735) ccw
  arc A177 (38.848, 38.8937) -> (38.848, 38.5763) centre (38.848, 38.735) ccw
  arc A178 (29.5021, 37.3063) -> (29.5021, 37.6238) centre (29.5021, 37.4651) ccw
  arc A179 (32.6644, 37.9413) -> (32.6644, 38.2587) centre (32.6644, 38.1) ccw
  arc A180 (84.2253, 37.9413) -> (84.2253, 38.2587) centre (84.2253, 38.1) ccw
  arc A181 (42.8914, 38.8937) -> (42.8914, 38.5763) centre (42.8914, 38.735) ccw
  arc A182 (25.0444, 38.5763) -> (25.0444, 38.8937) centre (25.0444, 38.735) ccw
  arc A183 (79.7179, 38.8937) -> (79.7179, 38.5763) centre (79.7179, 38.735) ccw
  arc A184 (25.6411, 39.2113) -> (25.6411, 39.5288) centre (25.6411, 39.37) ccw
  arc A185 (42.1064, 37.6238) -> (42.1064, 37.3063) centre (42.1064, 37.4651) ccw
  arc A186 (79.7179, 37.6238) -> (79.7179, 37.3063) centre (79.7179, 37.4651) ccw
  arc A187 (72.214, 38.8937) -> (72.214, 38.5763) centre (72.214, 38.735) ccw
  arc A188 (52.2664, 37.6238) -> (52.2664, 37.3063) centre (52.2664, 37.4651) ccw
  arc A189 (29.5021, 38.5763) -> (29.5021, 38.8937) centre (29.5021, 38.735) ccw
  arc A190 (72.517, 37.3063) -> (72.517, 37.6238) centre (72.517, 37.4651) ccw
  arc A191 (31.4579, 38.8937) -> (31.4579, 38.5763) centre (31.4579, 38.735) ccw
  arc A192 (39.1736, 38.5763) -> (39.1736, 38.8937) centre (39.1736, 38.735) ccw
  arc A193 (18.3143, 39.8463) -> (18.3143, 40.1638) centre (18.3143, 40.0051) ccw
  arc A194 (32.6644, 38.5763) -> (32.6644, 38.8937) centre (32.6644, 38.735) ccw
  arc A195 (40.9286, 39.8463) -> (40.9286, 40.1638) centre (40.9286, 40.0051) ccw
  arc A196 (5.4264, 39.5288) -> (5.4264, 39.2113) centre (5.4264, 39.37) ccw
  arc A197 (49.3141, 37.9413) -> (49.3141, 38.2587) centre (49.3141, 38.1) ccw
  arc A198 (27.5014, 40.7987) -> (27.5014, 40.4813) centre (27.5014, 40.64) ccw
  arc A199 (72.517, 39.2113) -> (72.517, 39.5288) centre (72.517, 39.37) ccw
  arc A200 (17.7419, 39.5288) -> (17.7419, 39.2113) centre (17.7419, 39.37) ccw
  arc A201 (31.4579, 40.1638) -> (31.4579, 39.8463) centre (31.4579, 40.0051) ccw
  arc A202 (4.5252, 40.7987) -> (4.5252, 40.4813) centre (4.5252, 40.64) ccw
  arc A203 (29.5021, 40.4813) -> (29.5021, 40.7987) centre (29.5021, 40.64) ccw
  arc A204 (35.3189, 39.5288) -> (35.3189, 39.2113) centre (35.3189, 39.37) ccw
  arc A205 (84.2253, 39.2113) -> (84.2253, 39.5288) centre (84.2253, 39.37) ccw
  arc A206 (39.8086, 39.2113) -> (39.8086, 39.5288) centre (39.8086, 39.37) ccw
  arc A207 (9.6052, 40.7987) -> (9.6052, 40.4813) centre (9.6052, 40.64) ccw
  arc A208 (31.4579, 40.7987) -> (31.4579, 40.4813) centre (31.4579, 40.64) ccw
  arc A209 (52.2859, 38.2587) -> (52.2859, 37.9413) centre (52.2859, 38.1) ccw
  arc A210 (72.517, 37.9413) -> (72.517, 38.2587) centre (72.517, 38.1) ccw
  arc A211 (17.7419, 40.1638) -> (17.7419, 39.8463) centre (17.7419, 40.0051) ccw
  arc A212 (26.148, 40.1638) -> (26.148, 39.8463) centre (26.148, 40.0051) ccw
  arc A213 (37.987, 40.4813) -> (37.987, 40.7987) centre (37.987, 40.64) ccw
  arc A214 (49.9686, 39.2113) -> (49.9686, 39.5288) centre (49.9686, 39.37) ccw
  arc A215 (4.7914, 40.1638) -> (4.7914, 39.8463) centre (4.7914, 40.0051) ccw
  arc A216 (37.352, 39.8463) -> (37.352, 40.1638) centre (37.352, 40.0051) ccw
  arc A217 (31.4579, 38.2587) -> (31.4579, 37.9413) centre (31.4579, 38.1) ccw
  arc A218 (79.7179, 39.5288) -> (79.7179, 39.2113) centre (79.7179, 39.37) ccw
  arc A219 (1.905, 39.8463) -> (1.905, 40.1638) centre (1.905, 40.0051) ccw
  arc A220 (0.7747, 40.1638) -> (0.7747, 39.8463) centre (0.7747, 40.0051) ccw
  arc A221 (72.214, 40.1638) -> (72.214, 39.8463) centre (72.214, 40.0051) ccw
  arc A222 (15.7861, 39.2113) -> (15.7861, 39.5288) centre (15.7861, 39.37) ccw
  arc A223 (18.1737, 40.4813) -> (18.1737, 40.7987) centre (18.1737, 40.64) ccw
  arc A224 (35.9986, 40.4813) -> (35.9986, 40.7987) centre (35.9986, 40.64) ccw
  arc A225 (39.483, 39.5288) -> (39.483, 39.2113) centre (39.483, 39.37) ccw
  arc A226 (0.7747, 38.8937) -> (0.7747, 38.5763) centre (0.7747, 38.735) ccw
  arc A227 (17.7419, 40.7987) -> (17.7419, 40.4813) centre (17.7419, 40.64) ccw
  arc A228 (29.5021, 39.2113) -> (29.5021, 39.5288) centre (29.5021, 39.37) ccw
  arc A229 (72.3737, 39.5288) -> (72.3737, 39.2113) centre (72.3737, 39.37) ccw
  arc A230 (50.5114, 40.1638) -> (50.5114, 39.8463) centre (50.5114, 40.0051) ccw
  arc A231 (37.6614, 40.7987) -> (37.6614, 40.4813) centre (37.6614, 40.64) ccw
  arc A232 (36.717, 39.2113) -> (36.717, 39.5288) centre (36.717, 39.37) ccw
  arc A233 (43.5264, 39.5288) -> (43.5264, 39.2113) centre (43.5264, 39.37) ccw
  arc A234 (42.1986, 41.1163) -> (42.1986, 41.4337) centre (42.1986, 41.275) ccw
  arc A235 (66.04, 41.4337) -> (66.04, 41.1163) centre (66.04, 41.275) ccw
  arc A236 (29.5021, 39.8463) -> (29.5021, 40.1638) centre (29.5021, 40.0051) ccw
  arc A237 (18.8428, 41.7513) -> (18.8428, 42.0688) centre (18.8428, 41.9101) ccw
  arc A238 (79.7179, 40.1638) -> (79.7179, 39.8463) centre (79.7179, 40.0051) ccw
  arc A239 (0.7747, 41.4337) -> (0.7747, 41.1163) centre (0.7747, 41.275) ccw
  arc A240 (38.2964, 41.4337) -> (38.2964, 41.1163) centre (38.2964, 41.275) ccw
  arc A241 (72.517, 39.8463) -> (72.517, 40.1638) centre (72.517, 40.0051) ccw
  arc A242 (60.2103, 40.4813) -> (60.2103, 40.7987) centre (60.2103, 40.64) ccw
  arc A243 (62.7503, 40.4813) -> (62.7503, 40.7987) centre (62.7503, 40.64) ccw
  arc A244 (51.6314, 40.7987) -> (51.6314, 40.4813) centre (51.6314, 40.64) ccw
  arc A245 (51.322, 39.8463) -> (51.322, 40.1638) centre (51.322, 40.0051) ccw
  arc A246 (31.4579, 39.5288) -> (31.4579, 39.2113) centre (31.4579, 39.37) ccw
  arc A247 (64.2497, 40.7987) -> (64.2497, 40.4813) centre (64.2497, 40.64) ccw
  arc A248 (72.517, 41.1163) -> (72.517, 41.4337) centre (72.517, 41.275) ccw
  arc A249 (5.0537, 41.4337) -> (5.0537, 41.1163) centre (5.0537, 41.275) ccw
  arc A250 (79.7179, 40.7987) -> (79.7179, 40.4813) centre (79.7179, 40.64) ccw
  arc A251 (42.1064, 41.4337) -> (42.1064, 41.1163) centre (42.1064, 41.275) ccw
  arc A252 (28.1364, 41.4337) -> (28.1364, 41.1163) centre (28.1364, 41.275) ccw
  arc A253 (59.1697, 40.7987) -> (59.1697, 40.4813) centre (59.1697, 40.64) ccw
  arc A254 (6.6508, 40.4813) -> (6.6508, 40.7987) centre (6.6508, 40.64) ccw
  arc A255 (72.517, 40.4813) -> (72.517, 40.7987) centre (72.517, 40.64) ccw
  arc A256 (56.9091, 41.1163) -> (56.9091, 41.4337) centre (56.9091, 41.275) ccw
  arc A257 (6.1223, 41.1163) -> (6.1223, 41.4337) centre (6.1223, 41.275) ccw
  arc A258 (15.7861, 40.4813) -> (15.7861, 40.7987) centre (15.7861, 40.64) ccw
  arc A259 (66.04, 41.1163) -> (66.04, 41.4337) centre (66.04, 41.275) ccw
  arc A260 (15.7861, 41.7513) -> (15.7861, 42.0688) centre (15.7861, 41.9101) ccw
  arc A261 (10.908, 41.4337) -> (10.908, 41.1163) centre (10.908, 41.275) ccw
  arc A262 (61.7097, 40.7987) -> (61.7097, 40.4813) centre (61.7097, 40.64) ccw
  arc A263 (15.7861, 41.1163) -> (15.7861, 41.4337) centre (15.7861, 41.275) ccw
  arc A264 (1.5708, 40.4813) -> (1.5708, 40.7987) centre (1.5708, 40.64) ccw
  arc A265 (1.0423, 41.1163) -> (1.0423, 41.4337) centre (1.0423, 41.275) ccw
  arc A266 (84.2253, 39.8463) -> (84.2253, 40.1638) centre (84.2253, 40.0051) ccw
  arc A267 (41.5636, 40.4813) -> (41.5636, 40.7987) centre (41.5636, 40.64) ccw
  arc A268 (5.1943, 42.0688) -> (5.1943, 41.7513) centre (5.1943, 41.9101) ccw
  arc A269 (0.7747, 40.7987) -> (0.7747, 40.4813) centre (0.7747, 40.64) ccw
  arc A270 (15.7861, 39.8463) -> (15.7861, 40.1638) centre (15.7861, 40.0051) ccw
  arc A271 (11.543, 42.0688) -> (11.543, 41.7513) centre (11.543, 41.9101) ccw
  arc A272 (84.2253, 40.4813) -> (84.2253, 40.7987) centre (84.2253, 40.64) ccw
  arc A273 (17.7419, 41.4337) -> (17.7419, 41.1163) centre (17.7419, 41.275) ccw
  arc A274 (35.3636, 41.1163) -> (35.3636, 41.4337) centre (35.3636, 41.275) ccw
  arc A275 (40.118, 40.1638) -> (40.118, 39.8463) centre (40.118, 40.0051) ccw
  arc A276 (41.4714, 40.7987) -> (41.4714, 40.4813) centre (41.4714, 40.64) ccw
  arc A277 (18.3143, 41.1163) -> (18.3143, 41.4337) centre (18.3143, 41.275) ccw
  arc A278 (66.04, 42.7037) -> (66.04, 42.3863) centre (66.04, 42.545) ccw
  arc A279 (81.28, 42.3863) -> (81.28, 42.7037) centre (81.28, 42.545) ccw
  arc A280 (39.1736, 42.3863) -> (39.1736, 42.7037) centre (39.1736, 42.545) ccw
  arc A281 (38.2964, 42.7037) -> (38.2964, 42.3863) centre (38.2964, 42.545) ccw
  arc A282 (28.1559, 42.0688) -> (28.1559, 41.7513) centre (28.1559, 41.9101) ccw
  arc A283 (31.4579, 41.4337) -> (31.4579, 41.1163) centre (31.4579, 41.275) ccw
  arc A284 (32.498, 42.7037) -> (32.498, 42.3863) centre (32.498, 42.545) ccw
  arc A285 (42.658, 42.7037) -> (42.658, 42.3863) centre (42.658, 42.545) ccw
  arc A286 (25.1841, 41.7513) -> (25.1841, 42.0688) centre (25.1841, 41.9101) ccw
  arc A287 (72.517, 41.7513) -> (72.517, 42.0688) centre (72.517, 41.9101) ccw
  arc A288 (57.6703, 40.4813) -> (57.6703, 40.7987) centre (57.6703, 40.64) ccw
  arc A289 (29.732, 42.3863) -> (29.732, 42.7037) centre (29.732, 42.545) ccw
  arc A290 (67.2068, 41.4337) -> (67.2068, 41.1163) centre (67.2068, 41.275) ccw
  arc A291 (0.9017, 41.7513) -> (0.9017, 42.0688) centre (0.9017, 41.9101) ccw
  arc A292 (29.5021, 41.7513) -> (29.5021, 42.0688) centre (29.5021, 41.9101) ccw
  arc A293 (79.7179, 42.0688) -> (79.7179, 41.7513) centre (79.7179, 41.9101) ccw
  arc A294 (31.863, 42.0688) -> (31.863, 41.7513) centre (31.863, 41.9101) ccw
  arc A295 (84.2253, 41.7513) -> (84.2253, 42.0688) centre (84.2253, 41.9101) ccw
  arc A296 (5.0537, 42.7037) -> (5.0537, 42.3863) centre (5.0537, 42.545) ccw
  arc A297 (13.3018, 42.3863) -> (13.3018, 42.7037) centre (13.3018, 42.545) ccw
  arc A298 (66.04, 42.3863) -> (66.04, 42.7037) centre (66.04, 42.545) ccw
  arc A299 (42.1259, 42.0688) -> (42.1259, 41.7513) centre (42.1259, 41.9101) ccw
  arc A300 (17.7419, 42.7037) -> (17.7419, 42.3863) centre (17.7419, 42.545) ccw
  arc A301 (0.7747, 42.7037) -> (0.7747, 42.3863) centre (0.7747, 42.545) ccw
  arc A302 (79.7179, 41.4337) -> (79.7179, 41.1163) centre (79.7179, 41.275) ccw
  arc A303 (52.2664, 41.4337) -> (52.2664, 41.1163) centre (52.2664, 41.275) ccw
  arc A304 (0.7747, 42.0688) -> (0.7747, 41.7513) centre (0.7747, 41.9101) ccw
  arc A305 (35.3441, 41.7513) -> (35.3441, 42.0688) centre (35.3441, 41.9101) ccw
  arc A306 (81.28, 42.7037) -> (81.28, 42.3863) centre (81.28, 42.545) ccw
  arc A307 (21.7972, 42.0688) -> (21.7972, 41.7513) centre (21.7972, 41.9101) ccw
  arc A308 (15.7861, 42.3863) -> (15.7861, 42.7037) centre (15.7861, 42.545) ccw
  arc A309 (1.0423, 42.3863) -> (1.0423, 42.7037) centre (1.0423, 42.545) ccw
  arc A310 (67.5513, 42.7037) -> (67.5513, 42.3863) centre (67.5513, 42.545) ccw
  arc A311 (5.9817, 41.7513) -> (5.9817, 42.0688) centre (5.9817, 41.9101) ccw
  arc A312 (66.04, 41.7513) -> (66.04, 42.0688) centre (66.04, 41.9101) ccw
  arc A313 (49.3336, 42.3863) -> (49.3336, 42.7037) centre (49.3336, 42.545) ccw
  arc A314 (38.3159, 42.0688) -> (38.3159, 41.7513) centre (38.3159, 41.9101) ccw
  arc A315 (84.2253, 41.1163) -> (84.2253, 41.4337) centre (84.2253, 41.275) ccw
  arc A316 (28.1364, 42.7037) -> (28.1364, 42.3863) centre (28.1364, 42.545) ccw
  arc A317 (52.4164, 42.0688) -> (52.4164, 41.7513) centre (52.4164, 41.9101) ccw
  arc A318 (56.6547, 41.7513) -> (56.6547, 42.0688) centre (56.6547, 41.9101) ccw
  arc A319 (29.5021, 41.1163) -> (29.5021, 41.4337) centre (29.5021, 41.275) ccw
  arc A320 (38.622, 41.1163) -> (38.622, 41.4337) centre (38.622, 41.275) ccw
  arc A321 (72.1491, 42.3863) -> (72.1491, 42.7037) centre (72.1491, 42.545) ccw
  arc A322 (39.1541, 41.7513) -> (39.1541, 42.0688) centre (39.1541, 41.9101) ccw
  arc A323 (12.178, 42.7037) -> (12.178, 42.3863) centre (12.178, 42.545) ccw
  arc A324 (66.04, 43.6563) -> (66.04, 43.9738) centre (66.04, 43.815) ccw
  arc A325 (43.293, 43.3387) -> (43.293, 43.0213) centre (43.293, 43.18) ccw
  arc A326 (17.7419, 43.3387) -> (17.7419, 43.0213) centre (17.7419, 43.18) ccw
  arc A327 (15.4025, 43.3387) -> (15.4025, 43.0213) centre (15.4025, 43.18) ccw
  arc A328 (14.6382, 42.7037) -> (14.6382, 42.3863) centre (14.6382, 42.545) ccw
  arc A329 (15.7861, 43.0213) -> (15.7861, 43.3387) centre (15.7861, 43.18) ccw
  arc A330 (25.2036, 42.3863) -> (25.2036, 42.7037) centre (25.2036, 42.545) ccw
  arc A331 (41.162, 43.6563) -> (41.162, 43.9738) centre (41.162, 43.815) ccw
  arc A332 (81.28, 43.6563) -> (81.28, 43.9738) centre (81.28, 43.815) ccw
  arc A333 (84.2253, 43.0213) -> (84.2253, 43.3387) centre (84.2253, 43.18) ccw
  arc A334 (66.04, 43.9738) -> (66.04, 43.6563) centre (66.04, 43.815) ccw
  arc A335 (27.5014, 43.3387) -> (27.5014, 43.0213) centre (27.5014, 43.18) ccw
  arc A336 (18.1737, 43.0213) -> (18.1737, 43.3387) centre (18.1737, 43.18) ccw
  arc A337 (35.9986, 43.0213) -> (35.9986, 43.3387) centre (35.9986, 43.18) ccw
  arc A338 (31.002, 43.6563) -> (31.002, 43.9738) centre (31.002, 43.815) ccw
  arc A339 (0.7747, 43.3387) -> (0.7747, 43.0213) centre (0.7747, 43.18) ccw
  arc A340 (35.3636, 42.3863) -> (35.3636, 42.7037) centre (35.3636, 42.545) ccw
  arc A341 (81.28, 43.0213) -> (81.28, 43.3387) centre (81.28, 43.18) ccw
  arc A342 (33.133, 43.3387) -> (33.133, 43.0213) centre (33.133, 43.18) ccw
  arc A343 (0.7747, 43.9738) -> (0.7747, 43.6563) centre (0.7747, 43.815) ccw
  arc A344 (49.9686, 43.0213) -> (49.9686, 43.3387) centre (49.9686, 43.18) ccw
  arc A345 (84.2253, 42.3863) -> (84.2253, 42.7037) centre (84.2253, 42.545) ccw
  arc A346 (81.28, 43.3387) -> (81.28, 43.0213) centre (81.28, 43.18) ccw
  arc A347 (1.0423, 43.6563) -> (1.0423, 43.9738) centre (1.0423, 43.815) ccw
  arc A348 (67.5513, 43.9738) -> (67.5513, 43.6563) centre (67.5513, 43.815) ccw
  arc A349 (6.1223, 42.3863) -> (6.1223, 42.7037) centre (6.1223, 42.545) ccw
  arc A350 (39.8086, 43.0213) -> (39.8086, 43.3387) centre (39.8086, 43.18) ccw
  arc A351 (18.3143, 42.3863) -> (18.3143, 42.7037) centre (18.3143, 42.545) ccw
  arc A352 (6.6508, 43.0213) -> (6.6508, 43.3387) centre (6.6508, 43.18) ccw
  arc A353 (4.5252, 43.3387) -> (4.5252, 43.0213) centre (4.5252, 43.18) ccw
  arc A354 (17.7419, 42.0688) -> (17.7419, 41.7513) centre (17.7419, 41.9101) ccw
  arc A355 (49.1836, 41.7513) -> (49.1836, 42.0688) centre (49.1836, 41.9101) ccw
  arc A356 (22.3257, 42.7037) -> (22.3257, 42.3863) centre (22.3257, 42.545) ccw
  arc A357 (17.7419, 43.9738) -> (17.7419, 43.6563) centre (17.7419, 43.815) ccw
  arc A358 (67.5178, 42.0688) -> (67.5178, 41.7513) centre (67.5178, 41.9101) ccw
  arc A359 (82.4468, 42.7037) -> (82.4468, 42.3863) centre (82.4468, 42.545) ccw
  arc A360 (40.118, 43.9738) -> (40.118, 43.6563) centre (40.118, 43.815) ccw
  arc A361 (22.4663, 43.3387) -> (22.4663, 43.0213) centre (22.4663, 43.18) ccw
  arc A362 (71.8947, 43.6563) -> (71.8947, 43.9738) centre (71.8947, 43.815) ccw
  arc A363 (22.3257, 43.9738) -> (22.3257, 43.6563) centre (22.3257, 43.815) ccw
  arc A364 (81.28, 43.9738) -> (81.28, 43.6563) centre (81.28, 43.815) ccw
  arc A365 (66.04, 42.0688) -> (66.04, 41.7513) centre (66.04, 41.9101) ccw
  arc A366 (25.8386, 43.0213) -> (25.8386, 43.3387) centre (25.8386, 43.18) ccw
  arc A367 (15.6337, 43.9738) -> (15.6337, 43.6563) centre (15.6337, 43.815) ccw
  arc A368 (81.28, 45.2437) -> (81.28, 44.9263) centre (81.28, 45.085) ccw
  arc A369 (0.7747, 44.6088) -> (0.7747, 44.2913) centre (0.7747, 44.4501) ccw
  arc A370 (15.762, 43.6563) -> (15.762, 43.9738) centre (15.762, 43.815) ccw
  arc A371 (81.28, 44.9263) -> (81.28, 45.2437) centre (81.28, 45.085) ccw
  arc A372 (21.7972, 44.6088) -> (21.7972, 44.2913) centre (21.7972, 44.4501) ccw
  arc A373 (66.04, 45.2437) -> (66.04, 44.9263) centre (66.04, 45.085) ccw
  arc A374 (17.7173, 44.6088) -> (17.7173, 44.2913) centre (17.7173, 44.4501) ccw
  arc A375 (82.7913, 43.9738) -> (82.7913, 43.6563) centre (82.7913, 43.815) ccw
  arc A376 (41.388, 45.2437) -> (41.388, 44.9263) centre (41.388, 45.085) ccw
  arc A377 (66.04, 44.6088) -> (66.04, 44.2913) centre (66.04, 44.4501) ccw
  arc A378 (1.5708, 43.0213) -> (1.5708, 43.3387) centre (1.5708, 43.18) ccw
  arc A379 (37.6614, 43.3387) -> (37.6614, 43.0213) centre (37.6614, 43.18) ccw
  arc A380 (10.047, 45.5613) -> (10.047, 45.8787) centre (10.047, 45.72) ccw
  arc A381 (6.6508, 45.5613) -> (6.6508, 45.8787) centre (6.6508, 45.72) ccw
  arc A382 (1.5708, 45.5613) -> (1.5708, 45.8787) centre (1.5708, 45.72) ccw
  arc A383 (18.3143, 43.6563) -> (18.3143, 43.9738) centre (18.3143, 43.815) ccw
  arc A384 (6.1223, 43.6563) -> (6.1223, 43.9738) centre (6.1223, 43.815) ccw
  arc A385 (66.04, 43.3387) -> (66.04, 43.0213) centre (66.04, 43.18) ccw
  arc A386 (40.753, 44.6088) -> (40.753, 44.2913) centre (40.753, 44.4501) ccw
  arc A387 (66.04, 44.2913) -> (66.04, 44.6088) centre (66.04, 44.4501) ccw
  arc A388 (23.5113, 45.5613) -> (23.5113, 45.8787) centre (23.5113, 45.72) ccw
  arc A389 (81.28, 44.6088) -> (81.28, 44.2913) centre (81.28, 44.4501) ccw
  arc A390 (41.797, 44.2913) -> (41.797, 44.6088) centre (41.797, 44.4501) ccw
  arc A391 (9.6052, 45.8787) -> (9.6052, 45.5613) centre (9.6052, 45.72) ccw
  arc A392 (67.2068, 45.2437) -> (67.2068, 44.9263) centre (67.2068, 45.085) ccw
  arc A393 (0.9017, 44.2913) -> (0.9017, 44.6088) centre (0.9017, 44.4501) ccw
  arc A394 (71.8947, 44.2913) -> (71.8947, 44.6088) centre (71.8947, 44.4501) ccw
  arc A395 (23.671, 44.9263) -> (23.671, 45.2437) centre (23.671, 45.085) ccw
  arc A396 (54.5937, 44.6088) -> (54.5937, 44.2913) centre (54.5937, 44.4501) ccw
  arc A397 (84.2253, 43.6563) -> (84.2253, 43.9738) centre (84.2253, 43.815) ccw
  arc A398 (5.0537, 43.9738) -> (5.0537, 43.6563) centre (5.0537, 43.815) ccw
  arc A399 (30.367, 43.0213) -> (30.367, 43.3387) centre (30.367, 43.18) ccw
  arc A400 (56.6547, 44.2913) -> (56.6547, 44.6088) centre (56.6547, 44.4501) ccw
  arc A401 (6.1223, 44.9263) -> (6.1223, 45.2437) centre (6.1223, 45.085) ccw
  arc A402 (1.0423, 44.9263) -> (1.0423, 45.2437) centre (1.0423, 45.085) ccw
  arc A403 (82.7578, 43.3387) -> (82.7578, 43.0213) centre (82.7578, 43.18) ccw
  arc A404 (82.7913, 45.2437) -> (82.7913, 44.9263) centre (82.7913, 45.085) ccw
  arc A405 (5.1943, 44.6088) -> (5.1943, 44.2913) centre (5.1943, 44.4501) ccw
  arc A406 (18.8428, 44.2913) -> (18.8428, 44.6088) centre (18.8428, 44.4501) ccw
  arc A407 (84.2253, 44.9263) -> (84.2253, 45.2437) centre (84.2253, 45.085) ccw
  arc A408 (71.8947, 43.0213) -> (71.8947, 43.3387) centre (71.8947, 43.18) ccw
  arc A409 (4.5252, 45.8787) -> (4.5252, 45.5613) centre (4.5252, 45.72) ccw
  arc A410 (67.5178, 44.6088) -> (67.5178, 44.2913) centre (67.5178, 44.4501) ccw
  arc A411 (31.637, 44.2913) -> (31.637, 44.6088) centre (31.637, 44.4501) ccw
  arc A412 (42.432, 44.9263) -> (42.432, 45.2437) centre (42.432, 45.085) ccw
  arc A413 (56.9091, 44.9263) -> (56.9091, 45.2437) centre (56.9091, 45.085) ccw
  arc A414 (66.04, 44.9263) -> (66.04, 45.2437) centre (66.04, 45.085) ccw
  arc A415 (5.0537, 45.2437) -> (5.0537, 44.9263) centre (5.0537, 45.085) ccw
  arc A416 (79.4897, 47.1487) -> (79.4897, 46.8313) centre (79.4897, 46.99) ccw
  arc A417 (54.434, 45.2437) -> (54.434, 44.9263) centre (54.434, 45.085) ccw
  arc A418 (71.8947, 45.5613) -> (71.8947, 45.8787) centre (71.8947, 45.72) ccw
  arc A419 (15.7603, 46.8313) -> (15.7603, 47.1487) centre (15.7603, 46.99) ccw
  arc A420 (84.2253, 46.8313) -> (84.2253, 47.1487) centre (84.2253, 46.99) ccw
  arc A421 (17.2597, 47.1487) -> (17.2597, 46.8313) centre (17.2597, 46.99) ccw
  arc A422 (9.9191, 47.4663) -> (9.9191, 47.7837) centre (9.9191, 47.625) ccw
  arc A423 (61.073, 47.1487) -> (61.073, 46.8313) centre (61.073, 46.99) ccw
  arc A424 (10.4521, 46.8313) -> (10.4521, 47.1487) centre (10.4521, 46.99) ccw
  arc A425 (84.2253, 45.5613) -> (84.2253, 45.8787) centre (84.2253, 45.72) ccw
  arc A426 (81.28, 46.1963) -> (81.28, 46.5138) centre (81.28, 46.3551) ccw
  arc A427 (84.2253, 44.2913) -> (84.2253, 44.6088) centre (84.2253, 44.4501) ccw
  arc A428 (62.7503, 45.5613) -> (62.7503, 45.8787) centre (62.7503, 45.72) ccw
  line L1 (15.353, 46.99) -> (15.7603, 46.99)
  arc A429 (15.988, 46.5138) -> (15.988, 46.1963) centre (15.988, 46.3551) ccw
  arc A430 (0.7747, 45.2437) -> (0.7747, 44.9263) centre (0.7747, 45.085) ccw
  arc A431 (71.8947, 44.9263) -> (71.8947, 45.2437) centre (71.8947, 45.085) ccw
  arc A432 (82.4468, 46.5138) -> (82.4468, 46.1963) centre (82.4468, 46.3551) ccw
  arc A433 (5.9817, 44.2913) -> (5.9817, 44.6088) centre (5.9817, 44.4501) ccw
  arc A434 (0.7747, 45.8787) -> (0.7747, 45.5613) centre (0.7747, 45.72) ccw
  arc A435 (17.258, 45.2437) -> (17.258, 44.9263) centre (17.258, 45.085) ccw
  arc A436 (76.9497, 47.1487) -> (76.9497, 46.8313) centre (76.9497, 46.99) ccw
  arc A437 (81.28, 45.8787) -> (81.28, 45.5613) centre (81.28, 45.72) ccw
  arc A438 (81.28, 46.5138) -> (81.28, 46.1963) centre (81.28, 46.3551) ccw
  arc A439 (80.9625, 48.1013) -> (80.9625, 48.4188) centre (80.9625, 48.2601) ccw
  arc A440 (71.247, 48.1013) -> (71.247, 48.4188) centre (71.247, 48.2601) ccw
  arc A441 (57.6703, 45.5613) -> (57.6703, 45.8787) centre (57.6703, 45.72) ccw
  arc A442 (74.2603, 48.1013) -> (74.2603, 48.4188) centre (74.2603, 48.2601) ccw
  arc A443 (74.4097, 47.1487) -> (74.4097, 46.8313) centre (74.4097, 46.99) ccw
  arc A444 (0.7747, 47.7837) -> (0.7747, 47.4663) centre (0.7747, 47.625) ccw
  arc A445 (59.1697, 45.8787) -> (59.1697, 45.5613) centre (59.1697, 45.72) ccw
  arc A446 (60.438, 47.7837) -> (60.438, 47.4663) centre (60.438, 47.625) ccw
  arc A447 (19.05, 47.7837) -> (19.05, 47.4663) centre (19.05, 47.625) ccw
  arc A448 (15.353, 47.1487) -> (15.353, 46.8313) centre (15.353, 46.99) ccw
  arc A449 (43.702, 46.1963) -> (43.702, 46.5138) centre (43.702, 46.3551) ccw
  arc A450 (42.658, 46.5138) -> (42.658, 46.1963) centre (42.658, 46.3551) ccw